Autodesk Inventor part; units mm, degrees
(part 2 of 2)
  arc A377 (-242.7, 447.09) -> (-236, 447.09) centre (-239.35, 447.09) ccw
  line L388 (-254.9, 447.09) -> (-254.9, 490.39)
  arc A378 (-248.2, 490.39) -> (-254.9, 490.39) centre (-251.55, 490.39) ccw
  line L389 (-248.2, 490.39) -> (-248.2, 447.09)
  arc A379 (-254.9, 447.09) -> (-248.2, 447.09) centre (-251.55, 447.09) ccw
  line L390 (-267.1, 447.09) -> (-267.1, 490.39)
  arc A380 (-260.4, 490.39) -> (-267.1, 490.39) centre (-263.75, 490.39) ccw
  line L391 (-260.4, 490.39) -> (-260.4, 447.09)
  arc A381 (-267.1, 447.09) -> (-260.4, 447.09) centre (-263.75, 447.09) ccw
  line L392 (-279.3, 447.09) -> (-279.3, 490.39)
  arc A382 (-272.6, 490.39) -> (-279.3, 490.39) centre (-275.95, 490.39) ccw
  line L393 (-272.6, 490.39) -> (-272.6, 447.09)
  arc A383 (-279.3, 447.09) -> (-272.6, 447.09) centre (-275.95, 447.09) ccw
  line L394 (-291.5, 447.09) -> (-291.5, 490.39)
  arc A384 (-284.8, 490.39) -> (-291.5, 490.39) centre (-288.15, 490.39) ccw
  line L395 (-284.8, 490.39) -> (-284.8, 447.09)
  arc A385 (-291.5, 447.09) -> (-284.8, 447.09) centre (-288.15, 447.09) ccw
  line L396 (-303.7, 447.09) -> (-303.7, 490.39)
  arc A386 (-297, 490.39) -> (-303.7, 490.39) centre (-300.35, 490.39) ccw
  line L397 (-297, 490.39) -> (-297, 447.09)
  arc A387 (-303.7, 447.09) -> (-297, 447.09) centre (-300.35, 447.09) ccw
  line L398 (-315.9, 447.09) -> (-315.9, 490.39)
  arc A388 (-309.2, 490.39) -> (-315.9, 490.39) centre (-312.55, 490.39) ccw
  line L399 (-309.2, 490.39) -> (-309.2, 447.09)
  arc A389 (-315.9, 447.09) -> (-309.2, 447.09) centre (-312.55, 447.09) ccw
  line L400 (-328.1, 447.09) -> (-328.1, 490.39)
  arc A390 (-321.4, 490.39) -> (-328.1, 490.39) centre (-324.75, 490.39) ccw
  line L401 (-321.4, 490.39) -> (-321.4, 447.09)
  arc A391 (-328.1, 447.09) -> (-321.4, 447.09) centre (-324.75, 447.09) ccw
  line L402 (-340.3, 447.09) -> (-340.3, 490.39)
  arc A392 (-333.6, 490.39) -> (-340.3, 490.39) centre (-336.95, 490.39) ccw
  line L403 (-333.6, 490.39) -> (-333.6, 447.09)
  arc A393 (-340.3, 447.09) -> (-333.6, 447.09) centre (-336.95, 447.09) ccw
  line L404 (-352.5, 447.09) -> (-352.5, 490.39)
  arc A394 (-345.8, 490.39) -> (-352.5, 490.39) centre (-349.15, 490.39) ccw
  line L405 (-345.8, 490.39) -> (-345.8, 447.09)
  arc A395 (-352.5, 447.09) -> (-345.8, 447.09) centre (-349.15, 447.09) ccw
  line L406 (-364.7, 447.09) -> (-364.7, 490.39)
  arc A396 (-358, 490.39) -> (-364.7, 490.39) centre (-361.35, 490.39) ccw
  line L407 (-358, 490.39) -> (-358, 447.09)
  arc A397 (-364.7, 447.09) -> (-358, 447.09) centre (-361.35, 447.09) ccw
  line L408 (-35.3, 507.09) -> (-35.3, 550.39)
  arc A398 (-28.6, 550.39) -> (-35.3, 550.39) centre (-31.95, 550.39) ccw
  line L409 (-28.6, 550.39) -> (-28.6, 507.09)
  arc A399 (-35.3, 507.09) -> (-28.6, 507.09) centre (-31.95, 507.09) ccw
  line L410 (-47.5, 507.09) -> (-47.5, 550.39)
  arc A400 (-40.8, 550.39) -> (-47.5, 550.39) centre (-44.15, 550.39) ccw
  line L411 (-40.8, 550.39) -> (-40.8, 507.09)
  arc A401 (-47.5, 507.09) -> (-40.8, 507.09) centre (-44.15, 507.09) ccw
  line L412 (-59.7, 507.09) -> (-59.7, 550.39)
  arc A402 (-53, 550.39) -> (-59.7, 550.39) centre (-56.35, 550.39) ccw
  line L413 (-53, 550.39) -> (-53, 507.09)
  arc A403 (-59.7, 507.09) -> (-53, 507.09) centre (-56.35, 507.09) ccw
  line L414 (-71.9, 507.09) -> (-71.9, 550.39)
  arc A404 (-65.2, 550.39) -> (-71.9, 550.39) centre (-68.55, 550.39) ccw
  line L415 (-65.2, 550.39) -> (-65.2, 507.09)
  arc A405 (-71.9, 507.09) -> (-65.2, 507.09) centre (-68.55, 507.09) ccw
  line L416 (-84.1, 507.09) -> (-84.1, 550.39)
  arc A406 (-77.4, 550.39) -> (-84.1, 550.39) centre (-80.75, 550.39) ccw
  line L417 (-77.4, 550.39) -> (-77.4, 507.09)
  arc A407 (-84.1, 507.09) -> (-77.4, 507.09) centre (-80.75, 507.09) ccw
  line L418 (-96.3, 507.09) -> (-96.3, 550.39)
  arc A408 (-89.6, 550.39) -> (-96.3, 550.39) centre (-92.95, 550.39) ccw
  line L419 (-89.6, 550.39) -> (-89.6, 507.09)
  arc A409 (-96.3, 507.09) -> (-89.6, 507.09) centre (-92.95, 507.09) ccw
  line L420 (-108.5, 507.09) -> (-108.5, 550.39)
  arc A410 (-101.8, 550.39) -> (-108.5, 550.39) centre (-105.15, 550.39) ccw
  line L421 (-101.8, 550.39) -> (-101.8, 507.09)
  arc A411 (-108.5, 507.09) -> (-101.8, 507.09) centre (-105.15, 507.09) ccw
  line L422 (-120.7, 507.09) -> (-120.7, 550.39)
  arc A412 (-114, 550.39) -> (-120.7, 550.39) centre (-117.35, 550.39) ccw
  line L423 (-114, 550.39) -> (-114, 507.09)
  arc A413 (-120.7, 507.09) -> (-114, 507.09) centre (-117.35, 507.09) ccw
  line L424 (-132.9, 507.09) -> (-132.9, 550.39)
  arc A414 (-126.2, 550.39) -> (-132.9, 550.39) centre (-129.55, 550.39) ccw
  line L425 (-126.2, 550.39) -> (-126.2, 507.09)
  arc A415 (-132.9, 507.09) -> (-126.2, 507.09) centre (-129.55, 507.09) ccw
  line L426 (-145.1, 507.09) -> (-145.1, 550.39)
  arc A416 (-138.4, 550.39) -> (-145.1, 550.39) centre (-141.75, 550.39) ccw
  line L427 (-138.4, 550.39) -> (-138.4, 507.09)
  arc A417 (-145.1, 507.09) -> (-138.4, 507.09) centre (-141.75, 507.09) ccw
  line L428 (-157.3, 507.09) -> (-157.3, 550.39)
  arc A418 (-150.6, 550.39) -> (-157.3, 550.39) centre (-153.95, 550.39) ccw
  line L429 (-150.6, 550.39) -> (-150.6, 507.09)
  arc A419 (-157.3, 507.09) -> (-150.6, 507.09) centre (-153.95, 507.09) ccw
  line L430 (-169.5, 507.09) -> (-169.5, 550.39)
  arc A420 (-162.8, 550.39) -> (-169.5, 550.39) centre (-166.15, 550.39) ccw
  line L431 (-162.8, 550.39) -> (-162.8, 507.09)
  arc A421 (-169.5, 507.09) -> (-162.8, 507.09) centre (-166.15, 507.09) ccw
  line L432 (-181.7, 507.09) -> (-181.7, 550.39)
  arc A422 (-175, 550.39) -> (-181.7, 550.39) centre (-178.35, 550.39) ccw
  line L433 (-175, 550.39) -> (-175, 507.09)
  arc A423 (-181.7, 507.09) -> (-175, 507.09) centre (-178.35, 507.09) ccw
  line L434 (-193.9, 507.09) -> (-193.9, 550.39)
  arc A424 (-187.2, 550.39) -> (-193.9, 550.39) centre (-190.55, 550.39) ccw
  line L435 (-187.2, 550.39) -> (-187.2, 507.09)
  arc A425 (-193.9, 507.09) -> (-187.2, 507.09) centre (-190.55, 507.09) ccw
  line L436 (-206.1, 507.09) -> (-206.1, 550.39)
  arc A426 (-199.4, 550.39) -> (-206.1, 550.39) centre (-202.75, 550.39) ccw
  line L437 (-199.4, 550.39) -> (-199.4, 507.09)
  arc A427 (-206.1, 507.09) -> (-199.4, 507.09) centre (-202.75, 507.09) ccw
  line L438 (-218.3, 507.09) -> (-218.3, 550.39)
  arc A428 (-211.6, 550.39) -> (-218.3, 550.39) centre (-214.95, 550.39) ccw
  line L439 (-211.6, 550.39) -> (-211.6, 507.09)
  arc A429 (-218.3, 507.09) -> (-211.6, 507.09) centre (-214.95, 507.09) ccw
  line L440 (-230.5, 507.09) -> (-230.5, 550.39)
  arc A430 (-223.8, 550.39) -> (-230.5, 550.39) centre (-227.15, 550.39) ccw
  line L441 (-223.8, 550.39) -> (-223.8, 507.09)
  arc A431 (-230.5, 507.09) -> (-223.8, 507.09) centre (-227.15, 507.09) ccw
  line L442 (-242.7, 507.09) -> (-242.7, 550.39)
  arc A432 (-236, 550.39) -> (-242.7, 550.39) centre (-239.35, 550.39) ccw
  line L443 (-236, 550.39) -> (-236, 507.09)
  arc A433 (-242.7, 507.09) -> (-236, 507.09) centre (-239.35, 507.09) ccw
  line L444 (-254.9, 507.09) -> (-254.9, 550.39)
  arc A434 (-248.2, 550.39) -> (-254.9, 550.39) centre (-251.55, 550.39) ccw
  line L445 (-248.2, 550.39) -> (-248.2, 507.09)
  arc A435 (-254.9, 507.09) -> (-248.2, 507.09) centre (-251.55, 507.09) ccw
  line L446 (-267.1, 507.09) -> (-267.1, 550.39)
  arc A436 (-260.4, 550.39) -> (-267.1, 550.39) centre (-263.75, 550.39) ccw
  line L447 (-260.4, 550.39) -> (-260.4, 507.09)
  arc A437 (-267.1, 507.09) -> (-260.4, 507.09) centre (-263.75, 507.09) ccw
  line L448 (-279.3, 507.09) -> (-279.3, 550.39)
  arc A438 (-272.6, 550.39) -> (-279.3, 550.39) centre (-275.95, 550.39) ccw
  line L449 (-272.6, 550.39) -> (-272.6, 507.09)
  arc A439 (-279.3, 507.09) -> (-272.6, 507.09) centre (-275.95, 507.09) ccw
  line L450 (-291.5, 507.09) -> (-291.5, 550.39)
  arc A440 (-284.8, 550.39) -> (-291.5, 550.39) centre (-288.15, 550.39) ccw
  line L451 (-284.8, 550.39) -> (-284.8, 507.09)
  arc A441 (-291.5, 507.09) -> (-284.8, 507.09) centre (-288.15, 507.09) ccw
  line L452 (-303.7, 507.09) -> (-303.7, 550.39)
  arc A442 (-297, 550.39) -> (-303.7, 550.39) centre (-300.35, 550.39) ccw
  line L453 (-297, 550.39) -> (-297, 507.09)
  arc A443 (-303.7, 507.09) -> (-297, 507.09) centre (-300.35, 507.09) ccw
  line L454 (-315.9, 507.09) -> (-315.9, 550.39)
  arc A444 (-309.2, 550.39) -> (-315.9, 550.39) centre (-312.55, 550.39) ccw
  line L455 (-309.2, 550.39) -> (-309.2, 507.09)
  arc A445 (-315.9, 507.09) -> (-309.2, 507.09) centre (-312.55, 507.09) ccw
  line L456 (-328.1, 507.09) -> (-328.1, 550.39)
  arc A446 (-321.4, 550.39) -> (-328.1, 550.39) centre (-324.75, 550.39) ccw
  line L457 (-321.4, 550.39) -> (-321.4, 507.09)
  arc A447 (-328.1, 507.09) -> (-321.4, 507.09) centre (-324.75, 507.09) ccw
  line L458 (-340.3, 507.09) -> (-340.3, 550.39)
  arc A448 (-333.6, 550.39) -> (-340.3, 550.39) centre (-336.95, 550.39) ccw
  line L459 (-333.6, 550.39) -> (-333.6, 507.09)
  arc A449 (-340.3, 507.09) -> (-333.6, 507.09) centre (-336.95, 507.09) ccw
  line L460 (-352.5, 507.09) -> (-352.5, 550.39)
  arc A450 (-345.8, 550.39) -> (-352.5, 550.39) centre (-349.15, 550.39) ccw
  line L461 (-345.8, 550.39) -> (-345.8, 507.09)
  arc A451 (-352.5, 507.09) -> (-345.8, 507.09) centre (-349.15, 507.09) ccw
  line L462 (-364.7, 507.09) -> (-364.7, 550.39)
  arc A452 (-358, 550.39) -> (-364.7, 550.39) centre (-361.35, 550.39) ccw
  line L463 (-358, 550.39) -> (-358, 507.09)
  arc A453 (-364.7, 507.09) -> (-358, 507.09) centre (-361.35, 507.09) ccw
  line L464 (-19.75, 383.74) -> (-19.75, 433.74) construction
  line L465 (-16.4, 387.09) -> (-16.4, 430.39)
  line L466 (-23.1, 430.39) -> (-23.1, 387.09)
  arc A454 (-23.1, 387.09) -> (-16.4, 387.09) centre (-19.75, 387.09) ccw
  arc A455 (-16.4, 430.39) -> (-23.1, 430.39) centre (-19.75, 430.39) ccw
  line L467 (-23.1, 490.39) -> (-23.1, 447.09)
  arc A456 (-16.4, 490.39) -> (-23.1, 490.39) centre (-19.75, 490.39) ccw
  line L468 (-16.4, 447.09) -> (-16.4, 490.39)
  arc A457 (-23.1, 447.09) -> (-16.4, 447.09) centre (-19.75, 447.09) ccw
  line L469 (-23.1, 550.39) -> (-23.1, 507.09)
  arc A458 (-16.4, 550.39) -> (-23.1, 550.39) centre (-19.75, 550.39) ccw
  line L470 (-16.4, 507.09) -> (-16.4, 550.39)
  arc A459 (-23.1, 507.09) -> (-16.4, 507.09) centre (-19.75, 507.09) ccw
  point P0 (-31.95, 288.74)
  point P1 (-19.75, 228.74)
  point P2 (-31.95, 348.74)
  point P3 (-19.75, 408.74)
  dimension "d43" = 50
  dimension "d47" = 12.2
  dimension "d50" = 60
  dimension "d62" = 60
  constraints: 938 end point, 928 point on circle, 696 symmetric about line, 460 centre point, 8 point on line, 8 tangent, 4 midpoint, 3 vertical, 2 parallel, 1 horizontal, 1360 other
  measures "d43" distance of L7.start L7.end
  measures "d47" distance of L8.start L10.start
  measures "d50" distance of L8.start L64.start
  measures "d62" distance of L234.start L235.start
extrude "Extrusión1" cut sketch "Boceto5" against normal blind 10
equation "\"d2\" = Grosor"
equation "\"d23\" = Anchura_desahogo_plegado"
equation "\"d25\" = Remanente_mínimo"
equation "\"d29\" = Radio_pliegue"
equation "\"d3\" = Anchura_desahogo_plegado"
equation "\"d4\" = Profundidad_desahogo_plegado"
equation "\"d5\" = Remanente_mínimo"
equation "\"d6\" = Radiodetransición"
equation "\"d9\" = Radio_pliegue"
equation "\"d10\" = Tamaño_destalonado"
equation "\"d11\" = TamañoSeparación"
equation "\"d12\" = Tamaño_de_radio_de_Jacobi"
equation "\"d13\" = Anchura_desahogo_plegado"
equation "\"d14\" = Profundidad_desahogo_plegado"
equation "\"d15\" = Remanente_mínimo"
equation "\"d16\" = Radiodetransición"
equation "\"d19\" = Radio_pliegue"
equation "\"d20\" = Tamaño_destalonado"
equation "\"d21\" = TamañoSeparación"
equation "\"d22\" = Tamaño_de_radio_de_Jacobi"
equation "\"d24\" = Profundidad_desahogo_plegado"
equation "\"d26\" = Radiodetransición"
equation "\"d30\" = Tamaño_destalonado"
equation "\"d31\" = TamañoSeparación"
equation "\"d32\" = Tamaño_de_radio_de_Jacobi"
equation "\"Radio_pliegue\" = Grosor"
equation "\"Anchura_desahogo_plegado\" = Grosor"
equation "\"Profundidad_desahogo_plegado\" = 0.5 * Grosor"
equation "\"Tamaño_destalonado\" = 4 * Grosor"
equation "\"Remanente_mínimo\" = 2 * Grosor"
equation "\"Radiodetransición\" = Radio_pliegue"
equation "\"Tamaño_de_radio_de_Jacobi\" = Radio_pliegue"
equation "\"TamañoSeparación\" = Grosor"
equation "\"Grosor\" = 0.5"
